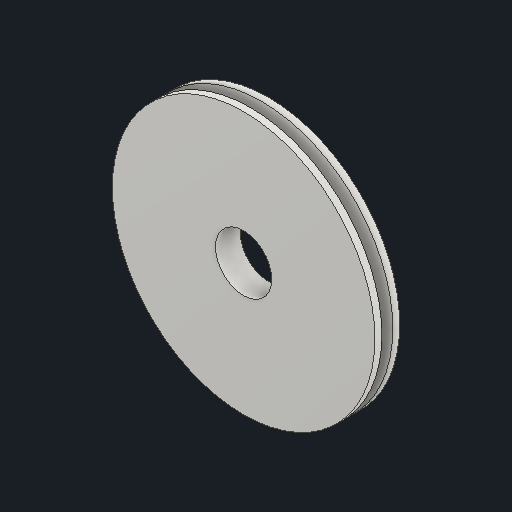
# Autodesk Inventor part: Poulie à gorge1
Saved by Autodesk Inventor 2026.2 (Build 302298010, 298A)
## iProperties
CustomPartVersion: 1
Created: 2026-03-31
Part Number: Poulie à gorge1
Material: Steel
Document SubType Name: Modeling
Designer: romai
Density: 1 g/cm^3
Appearance: Steel
Author: romai
Autodesk Inventor part; units mm, degrees
note: some values were not read from the file. Chosen so that the rebuilt part matches the saved one: direction of "Perçage1".
ref_plane "YZ Plane" through (0, 0, 0) normal (1, 0, 0) x (0, 1, 0)
ref_plane "XZ Plane" through (0, 0, 0) normal (0, 1, 0) x (-1, 0, 0)
sketch "Esquisse principale" plane through (0, 0, 0) normal (1, 0, 0) x (0, 1, 0)
  line L0 (0, 22) -> (116.5, 22)
  line L1 (116.5, 22) -> (116.5, 15.8615)
  line L2 (116.5, 15.8615) -> (105.5, 12.4984)
  line L3 (105.5, 12.4984) -> (105.5, 9.5016)
  line L4 (105.5, 9.5016) -> (116.5, 6.1385)
  line L5 (116.5, 6.1385) -> (116.5, 0)
  line L6 (116.5, 0) -> (0, 0)
  line L7 (114.5, 15.25) -> (114.5, 6.75) construction
  line L8 (105.5, 11) -> (114.5, 11) construction
  line L9 (116.5, 15.8615) -> (116.5, 6.1385)
  line L10 (0, -3.2) -> (0, 19.2) projected
  line L11 (0, 0) -> (0, 22)
  dimension "d0" = 8.5
  dimension "d1" = 34
  dimension "d2" = 2
  dimension "d6" = 22
  dimension "d21" = 229
  dimension "d25" = 11
  dimension "d27" = 11
  constraints: 22 end point, 5 perpendicular, 2 collinear, 2 midpoint, 2 point on line, 1 parallel
  measures "d0" distance of L7.start L7.end
  measures "d1" angle of L2 L4
  measures "d2" distance between parallel lines of L1 L7
  measures "d6" distance between parallel lines of L6 L0
  measures "d21" diameter of L7 L10
  measures "d25" distance between parallel lines of L3 L9
  measures "d27" distance between parallel lines of L6 L8
ref_plane "Plan de courroie" through (0, 105.5, 11) normal (0, 0, 1) x (1, 0, 0)
revolve "Corps" add sketch "Esquisse principale" angle 360 about axis through (0, 0, -10) along (0, 0, 1)
revolve "Bord" cut sketch "Esquisse principale" angle 360 about axis through (0, 0, -10) along (0, 0, 1) contours L9 L4 L3 L2
fillet "Congé externe" [suppressed]
fillet "Congé interne" [suppressed]
pattern_of_one "Réseau de bords"
sketch "Esquisse2" plane through (0, 0, 22) normal (0, 0, 1) x (1, 0, 0)
  circle A0 centre (0, 0) radius 116.5 projected
  constraints: 1 coincident
hole "Perçage1" at (0, 0, 22) direction (0, 0, -1) diameter 50 depth 22
equation "\"d0\" = da_Bw"
equation "\"d1\" = da_Alfa"
equation "\"d2\" = da_c"
equation "\"d21\" = da_Dw"
equation "\"d25\" = da_Hd"
equation "\"d27\" = da_Se"
equation "\"da_r1\" = 0"
equation "\"da_r2\" = 0"
equation "\"d18\" = da_Sg"
equation "\"d5\" = da_Se"
equation "\"da_Bw\" = 8.5"
equation "\"da_Alfa\" = 34deg"
equation "\"da_c\" = 2"
equation "\"da_Dw\" = 229"
equation "\"da_Hd\" = 11"
equation "\"da_Se\" = 11"
equation "\"da_Sg\" = 12"
body "Solid1"
